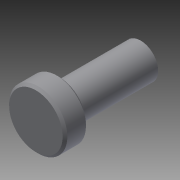
# Autodesk Inventor part: tappino
Saved by Autodesk Inventor 2015 (Build 190159000, 159)
## iProperties
Created: 2016-05-04
Part Number: tappino
Material: Generico
Document SubType Name: Modeling
Designer: galpama
Density: 1 g/cm^3
Appearance: Default
Author: galpama
Autodesk Inventor part; units mm, degrees
ref_plane "YZ Plane" through (0, 0, 0) normal (1, 0, 0) x (0, 1, 0)
ref_plane "XZ Plane" through (0, 0, 0) normal (0, 1, 0) x (-1, 0, 0)
ref_plane "XY Plane" through (0, 0, 0) normal (0, 0, 1) x (1, 0, 0)
sketch "Schizzo1" plane through (0, 0, 0) normal (0, 0, 1) x (1, 0, 0)
  line L0 (0, 0) -> (2.5, 0)
  line L1 (2.5, 0) -> (2.5, 2)
  line L2 (2.5, 2) -> (1.5, 2)
  line L3 (1.5, 2) -> (1.5, 9)
  line L4 (0, -0.9086) -> (0, 9.2919) construction
  line L5 (0, 9.2919) -> (0, 0)
  line L6 (0, 4.2303) -> (0, -9.1225) construction
  line L7 (0, 6.4019) -> (0, -8.8997) construction
  line L8 (0, 5.2919) -> (0, -9.4587) construction
  arc A0 (1.5, 9) -> (0, 9.2919) centre (0, 5.2919) ccw
  line L9 (0, 5.2919) -> (0, -13.4736) construction
  dimension "d0" = 2.5
  dimension "d1" = 2
  dimension "d7" = 1.5
  dimension "d16" = 2
  dimension "d18" = 8
  dimension "d19" = 7
  dimension "d20" = 9.2919
  constraints: 20 end point, 4 collinear, 2 point on circle, 1 centre point
  measures "d0" distance of L0.start L0.end
  measures "d1" distance of L0.end L1.end
  measures "d7" distance between parallel lines of L3 L4
  measures "d16" distance from line of L0 L2.end
  measures "d18" diameter of A0
  measures "d19" distance from line of L3.end L2
  measures "d20" distance from line of L0 L4.end
revolve "Rivoluzione1" add sketch "Schizzo1" angle 360 about axis through (0, -0.9086, 0) along (0, 1, 0)
chamfer "Smusso1" distance 0.2 angle 45 2 edges at (-2.5, 2, 0) (-2.5, 0, 0)
